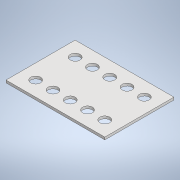
# Autodesk Inventor part: Lift.04.00.00.01
Saved by Autodesk Inventor 2021 (Build 250183000, 183)
## iProperties
Created: 2020-09-20
Part Number: Lift.04.00.00.01
Material: Типовые
Document SubType Name: ЛистМат
Designer: Kostya
Density: 1 g/cm^3
Sheet Metal Rule: По умолчанию_мм
Appearance: По умолчанию
Author: Kostya
Autodesk Inventor part; units mm, degrees
ref_plane "YZ Plane" through (0, 0, 0) normal (1, 0, 0) x (0, 1, 0)
ref_plane "XZ Plane" through (0, 0, 0) normal (0, 1, 0) x (-1, 0, 0)
ref_plane "XY Plane" through (0, 0, 0) normal (0, 0, 1) x (1, 0, 0)
sketch "Эскиз1" plane through (0, 0, 0) normal (0, 1, 0) x (-1, 0, 0)
  line L0 (-100, -70) -> (100, -70)
  line L1 (100, -70) -> (100, 70)
  line L2 (100, 70) -> (-100, 70)
  line L3 (-100, 70) -> (-100, -70)
  line L4 (-100, -70) -> (100, 70) construction
  line L5 (100, -70) -> (-100, 70) construction
  circle A0 centre (70, 40) radius 10
  circle A1 centre (70, -40) radius 10
  circle A2 centre (35, 40) radius 10
  circle A3 centre (35, -40) radius 10
  circle A4 centre (0, 40) radius 10
  circle A5 centre (0, -40) radius 10
  circle A6 centre (-35, 40) radius 10
  circle A7 centre (-35, -40) radius 10
  circle A8 centre (-70, 40) radius 10
  circle A9 centre (-70, -40) radius 10
  point P0 (0, 0)
  dimension "d0" = 200
  dimension "d1" = 140
  dimension "d2" = 30
  dimension "d3" = 30
  dimension "d4" = 20
  dimension "d7" = 80
  dimension "d10" = 35
  measures "d0" distance of L2.end L1.end
  measures "d1" distance of L1.end L0.end
  measures "d2" distance from line of L1 A0.centre
  measures "d3" distance from line of L2 A0.centre
  measures "d4" diameter of A0
  measures "d7" distance of A0.centre A1.centre
  measures "d10" distance of A0.centre A2.centre
extrude "Пластина1" add sketch "Эскиз1" along normal blind 5
equation "\"d13\" = Толщина"
equation "\"Радиус_гибки\" = Толщина"
equation "\"Ширина_просечки\" = Толщина"
equation "\"Глубина_просечки\" = 0.5 * Толщина"
equation "\"Радиус_перехода\" = Радиус_гибки"
equation "\"Радиус_Якоби\" = Радиус_гибки"
equation "\"Размер_зазора\" = Толщина"
equation "\"Толщина\" = 5"
